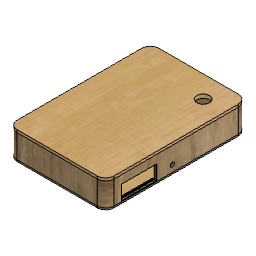
Wildfire prediction Device Full (Autodesk Fusion 360 design; units mm, degrees)
Autodesk Fusion 360 part; units mm, degrees
note: some values were not read from the file. Set by a fixed rule: which sketch regions a step uses.
(part 1 of 2)
sketch "PCB_wildfire-prediction-system_2026-03-05" plane through (0, 0, 0) normal (0, 0, 1) x (1, 0, 0)
  line L0 (72.8848, 47.7095) -> (75.6366, 50.4613)
  line L1 (75.6366, 56.1675) -> (78.2188, 58.7496)
  line L2 (75.6366, 50.4613) -> (75.6366, 56.1675)
  line L3 (93.0849, 97.6657) -> (85.1296, 89.7104)
  line L4 (85.1296, 60.3265) -> (83.9338, 59.1306)
  line L5 (85.1296, 89.7104) -> (85.1296, 60.3265)
  line L6 (79.3633, 25.6026) -> (79.2348, 25.6026)
  line L7 (80.6432, 26.8825) -> (79.3633, 25.6026)
  line L8 (80.6432, 45.1492) -> (80.6432, 26.8825)
  line L9 (78.0918, 47.7006) -> (80.6432, 45.1492)
  line L10 (79.2348, 13.8175) -> (79.2348, 23.0626)
  line L11 (82.5368, 10.5155) -> (79.2348, 13.8175)
  line L12 (83.9338, 61.6706) -> (83.9338, 62.8647)
  line L13 (78.0847, 97.6657) -> (78.0847, 72.6655)
  line L14 (76.5114, 29.9295) -> (72.8848, 29.9295)
  line L15 (79.6288, 33.0469) -> (76.5114, 29.9295)
  line L16 (78.0918, 45.1606) -> (79.6288, 43.6237)
  line L17 (79.6288, 43.6237) -> (79.6288, 33.0469)
  line L18 (76.5114, 25.786) -> (79.2348, 23.0626)
  line L19 (76.5114, 29.9295) -> (76.5114, 25.786)
  line L20 (60.0786, 69.2292) -> (57.3151, 66.4656)
  line L21 (78.0847, 69.2292) -> (60.0786, 69.2292)
  line L22 (78.0847, 68.7138) -> (78.0847, 69.2292)
  line L23 (83.9338, 62.8647) -> (78.0847, 68.7138)
  line L24 (78.0847, 69.2292) -> (78.0847, 72.6655)
  line L25 (72.3605, 36.2795) -> (71.6135, 37.0265)
  line L26 (76.8307, 36.2795) -> (72.3605, 36.2795)
  line L27 (71.6135, 37.0265) -> (71.6135, 54.0582)
  line L28 (78.0918, 37.5406) -> (76.8307, 36.2795)
  line L29 (71.6135, 54.0582) -> (72.8848, 55.3295)
  line L30 (83.9338, 54.0506) -> (81.9043, 54.0506)
  line L31 (74.1909, 41.3956) -> (72.8848, 40.0895)
  line L32 (81.9043, 54.0506) -> (74.1909, 46.3371)
  line L33 (74.1909, 46.3371) -> (74.1909, 41.3956)
  line L34 (24.2753, 76.6251) -> (24.2753, 60.759)
  line L35 (24.2753, 60.759) -> (50.0248, 35.0095)
  line L36 (18.1478, 82.7526) -> (24.2753, 76.6251)
  line L37 (27.021, 60.5533) -> (50.0248, 37.5495)
  line L38 (27.021, 76.4194) -> (27.021, 60.5533)
  line L39 (18.1478, 85.2926) -> (27.021, 76.4194)
  line L40 (51.3293, 31.9107) -> (51.3293, 43.865)
  line L41 (49.4325, 31.1995) -> (50.6181, 31.1995)
  line L42 (41.6428, 4.3936) -> (41.6428, 23.4098)
  line L43 (41.6428, 23.4098) -> (49.4325, 31.1995)
  line L44 (50.6181, 31.1995) -> (51.3293, 31.9107)
  line L45 (51.3293, 43.865) -> (50.0248, 45.1695)
  line L46 (50.5173, 26.1195) -> (49.3784, 26.1195)
  line L47 (51.8815, 27.4837) -> (50.5173, 26.1195)
  line L48 (50.0248, 47.7095) -> (51.8815, 45.8528)
  line L49 (51.8815, 45.8528) -> (51.8815, 27.4837)
  line L50 (49.3784, 26.1195) -> (44.1828, 20.9239)
  line L51 (44.1828, 20.9239) -> (44.1828, 4.3936)
  line L52 (59.8551, 60.0798) -> (50.0248, 50.2495)
  line L53 (59.8551, 66.4656) -> (59.8551, 60.0798)
  line L54 (93.0849, 27.6638) -> (93.0849, 72.6655)
  line L55 (82.5368, 17.1157) -> (93.0849, 27.6638)
  line L56 (-0.1656, 4.5206) -> (-0.1656, 98.5006)
  line L57 (97.6244, 0.7106) -> (3.6444, 0.7106)
  line L58 (101.4344, 98.5006) -> (101.4344, 4.5206)
  line L59 (3.6444, 102.3106) -> (97.6244, 102.3106)
  arc A0 (101.4344, 98.5006) -> (97.6244, 102.3106) centre (97.6244, 98.5006) ccw
  arc A1 (97.6244, 0.7106) -> (101.4344, 4.5206) centre (97.6244, 4.5206) ccw
  arc A2 (-0.1656, 4.5206) -> (3.6444, 0.7106) centre (3.6444, 4.5206) ccw
  arc A3 (3.6444, 102.3106) -> (-0.1656, 98.5006) centre (3.6444, 98.5006) ccw
  line L60 (76.3049, 61.2896) -> (72.8848, 57.8695)
  line L61 (78.2188, 61.2896) -> (76.3049, 61.2896)
  line L62 (45.5572, 56.3242) -> (45.5572, 52.8619)
  line L63 (45.5572, 52.8619) -> (49.4381, 48.981)
  line L64 (46.4688, 57.2358) -> (45.5572, 56.3242)
  line L65 (66.5333, 48.981) -> (72.8848, 42.6295)
  line L66 (49.4381, 48.981) -> (66.5333, 48.981)
  line L67 (54.976, 43.8995) -> (49.325, 43.8995)
  line L68 (74.2716, 42.1599) -> (73.4713, 41.3595)
  line L69 (72.8848, 45.1695) -> (72.8848, 44.6902)
  line L70 (49.325, 43.8995) -> (45.1165, 48.108)
  line L71 (57.516, 41.3595) -> (54.976, 43.8995)
  line L72 (73.4713, 41.3595) -> (57.516, 41.3595)
  line L73 (45.1165, 58.3836) -> (46.4688, 59.7359)
  line L74 (72.8848, 44.6902) -> (74.2716, 43.3034)
  line L75 (45.1165, 48.108) -> (45.1165, 58.3836)
  line L76 (74.2716, 43.3034) -> (74.2716, 42.1599)
  line L77 (74.8983, 31.1995) -> (77.9551, 28.1426)
  line L78 (50.0248, 42.6295) -> (61.4548, 31.1995)
  line L79 (61.4548, 31.1995) -> (74.8983, 31.1995)
  line L80 (79.2348, 28.1426) -> (77.9551, 28.1426)
  line L81 (73.532, 46.4395) -> (72.3562, 46.4395)
  line L82 (78.0918, 40.0806) -> (74.5457, 43.6267)
  line L83 (74.5457, 45.4258) -> (73.532, 46.4395)
  line L84 (74.5457, 43.6267) -> (74.5457, 45.4258)
  line L85 (72.3562, 46.4395) -> (71.5787, 47.217)
  line L86 (71.5787, 51.4834) -> (72.8848, 52.7895)
  line L87 (71.5787, 47.217) -> (71.5787, 51.4834)
  line L88 (78.0918, 42.6206) -> (75.9592, 44.7532)
  line L89 (75.9592, 44.7532) -> (75.9592, 47.1751)
  line L90 (75.9592, 47.1751) -> (72.8848, 50.2495)
  line L91 (78.0918, 47.7006) -> (78.0918, 49.1073)
  line L92 (78.4728, 53.6696) -> (78.2188, 53.6696)
  line L93 (83.9338, 59.1306) -> (78.4728, 53.6696)
  line L94 (78.2188, 53.6696) -> (78.2188, 49.2343)
  line L95 (78.2188, 49.2343) -> (78.0918, 49.1073)
  line L96 (57.5737, 6.0441) -> (77.1322, 25.6026)
  line L97 (38.2133, 6.0441) -> (57.5737, 6.0441)
  line L98 (77.1322, 25.6026) -> (79.2348, 25.6026)
  line L99 (36.5628, 4.3936) -> (38.2133, 6.0441)
  line L100 (85.1296, 60.3265) -> (83.9338, 59.1306)
  line L101 (64.9351, 66.4656) -> (67.2272, 64.1735)
  line L102 (85.1296, 62.7867) -> (85.1296, 60.3265)
  line L103 (83.7428, 64.1735) -> (85.1296, 62.7867)
  line L104 (67.2272, 64.1735) -> (83.7428, 64.1735)
  line L105 (18.1478, 80.2126) -> (47.9202, 80.2126)
  line L106 (47.9202, 80.2126) -> (61.1251, 67.0077)
  line L107 (64.9351, 66.4656) -> (63.576, 67.8248)
  line L108 (63.576, 67.8248) -> (61.9422, 67.8248)
  line L109 (61.9422, 67.8248) -> (61.1251, 67.0077)
  line L110 (49.7591, 59.5708) -> (48.2615, 58.0732)
  line L111 (46.6537, 55.9858) -> (46.4688, 55.9858)
  line L112 (61.1251, 65.9317) -> (54.7642, 59.5708)
  line L113 (48.2615, 57.5937) -> (46.6537, 55.9858)
  line L114 (48.2615, 58.0732) -> (48.2615, 57.5937)
  line L115 (61.1251, 67.0077) -> (61.1251, 65.9317)
  line L116 (54.7642, 59.5708) -> (49.7591, 59.5708)
  line L117 (83.9338, 61.6706) -> (82.7397, 61.6706)
  line L118 (82.5368, 10.5155) -> (83.4367, 10.5155)
  line L119 (83.4367, 10.5155) -> (87.0369, 14.1157)
  line L120 (82.7397, 61.6706) -> (82.7397, 60.7306)
  line L121 (82.7397, 60.7306) -> (78.2188, 56.2096)
  line L122 (76.4946, 54.4855) -> (76.4946, 46.5713)
  line L123 (78.2188, 56.2096) -> (76.4946, 54.4855)
  line L124 (76.4946, 46.5713) -> (77.9054, 45.1606)
  line L125 (77.9054, 45.1606) -> (78.0918, 45.1606)
  line L126 (35.4536, 2.9628) -> (34.0228, 4.3936)
  line L127 (37.672, 2.9628) -> (35.4536, 2.9628)
  line L128 (39.1028, 4.3936) -> (37.672, 2.9628)
  line L129 (39.1028, 4.3936) -> (40.5194, 2.9771)
  line L130 (40.5194, 2.9771) -> (74.9983, 2.9771)
  line L131 (74.9983, 2.9771) -> (82.5368, 10.5155)
  line L132 (57.3151, 66.4656) -> (53.9417, 63.0923)
  line L133 (53.9417, 63.0923) -> (46.4688, 63.0923)
  line L134 (46.4688, 62.2355) -> (46.4688, 63.0923)
  line L135 (18.1478, 77.6726) -> (31.8884, 77.6726)
  line L136 (31.8884, 77.6726) -> (46.4688, 63.0923)
  line L137 (78.7583, 36.2434) -> (74.1909, 36.2434)
  line L138 (83.9338, 56.5906) -> (79.5747, 52.2315)
  line L139 (79.5747, 52.2315) -> (79.5747, 37.0598)
  line L140 (79.5747, 37.0598) -> (78.7583, 36.2434)
  line L141 (74.1909, 36.2434) -> (72.8848, 37.5495)
  line L142 (62.3951, 65.1598) -> (50.0248, 52.7895)
  line L143 (62.3951, 66.4656) -> (62.3951, 65.1598)
  line L144 (47.7387, 63.8297) -> (47.7387, 52.0187)
  line L145 (44.4367, 63.8297) -> (47.7387, 63.8297)
  line L146 (44.4367, 51.8917) -> (44.4367, 63.8297)
  line L147 (47.7387, 51.8917) -> (44.4367, 51.8917)
  line L148 (2.8371, 13.6149) -> (40.838, 13.6149)
  line L149 (40.838, 63.6148) -> (2.8371, 63.6148)
  line L150 (40.838, 13.6149) -> (40.838, 63.6148)
  line L151 (2.8371, 63.6148) -> (2.8371, 13.6149)
  line L152 (42.8378, 19.6157) -> (40.838, 19.6157)
  line L153 (42.8378, 19.6157) -> (42.8378, 38.6158)
  line L154 (42.8378, 38.6158) -> (40.838, 38.6158)
  line L155 (2.8371, 36.1167) -> (0.3378, 36.1167)
  line L156 (0.3378, 21.1156) -> (2.8371, 21.1156)
  line L157 (2.8379, 36.1156) -> (2.8371, 36.1167)
  line L158 (0.3378, 36.1167) -> (0.3378, 21.1156)
  line L159 (91.4626, 33.3886) -> (91.4626, 19.0376)
  line L160 (91.4626, 19.0376) -> (76.4847, 19.0376)
  line L161 (76.4847, 19.0376) -> (76.4847, 33.3886)
  line L162 (76.4847, 33.3886) -> (91.4626, 33.3886)
  line L163 (48.7548, 62.8698) -> (74.1548, 62.8698)
  line L164 (48.7548, 2.8696) -> (48.7548, 62.8698)
  line L165 (74.1548, 62.8698) -> (74.1548, 2.8696)
  line L166 (74.1548, 2.8696) -> (48.7548, 2.8696)
  line L167 (56.8109, 96.1056) -> (54.1109, 96.1056)
  line L168 (56.8109, 98.7056) -> (56.8109, 96.1056)
  line L169 (54.1109, 96.1056) -> (54.1109, 98.7056)
  line L170 (54.1109, 98.7056) -> (56.8109, 98.7056)
  line L171 (47.8209, 100.4056) -> (47.8209, 64.8057)
  line L172 (73.9008, 64.8057) -> (73.9008, 100.4056)
  line L173 (47.8209, 64.8057) -> (73.9008, 64.8057)
  line L174 (73.9008, 100.4056) -> (47.8209, 100.4056)
  line L175 (32.4988, 2.6156) -> (32.4988, 6.1716)
  line L176 (45.7068, 2.6156) -> (32.4988, 2.6156)
  line L177 (32.4988, 6.1716) -> (45.7068, 6.1716)
  line L178 (45.7068, 6.1716) -> (45.7068, 2.6156)
  line L179 (77.3298, 43.8906) -> (76.8218, 44.3986)
  line L180 (77.3298, 41.3506) -> (76.8218, 41.8586)
  line L181 (76.8218, 43.3826) -> (77.3298, 43.8906)
  line L182 (76.8218, 46.9386) -> (76.8218, 48.9706)
  line L183 (76.8218, 39.3186) -> (76.8218, 40.8426)
  line L184 (76.8218, 36.2706) -> (76.8218, 38.3026)
  line L185 (76.8218, 41.8586) -> (76.8218, 43.3826)
  line L186 (76.8218, 38.3026) -> (77.3298, 38.8106)
  line L187 (79.3618, 38.3026) -> (79.3618, 36.2706)
  line L188 (78.8538, 43.8906) -> (79.3618, 43.3826)
  line L189 (76.8218, 45.9226) -> (77.3298, 46.4306)
  line L190 (79.3618, 44.3986) -> (78.8538, 43.8906)
  line L191 (79.3618, 40.8426) -> (79.3618, 39.3186)
  line L192 (79.3618, 41.8586) -> (78.8538, 41.3506)
  line L193 (79.3618, 43.3826) -> (79.3618, 41.8586)
  line L194 (76.8218, 48.9706) -> (79.3618, 48.9706)
  line L195 (76.8218, 44.3986) -> (76.8218, 45.9226)
  line L196 (77.3298, 38.8106) -> (76.8218, 39.3186)
  line L197 (78.8538, 46.4306) -> (79.3618, 45.9226)
  line L198 (77.3298, 46.4306) -> (76.8218, 46.9386)
  line L199 (79.3618, 48.9706) -> (79.3618, 46.9386)
  line L200 (79.3618, 36.2706) -> (76.8218, 36.2706)
  line L201 (76.8218, 40.8426) -> (77.3298, 41.3506)
  line L202 (79.3618, 46.9386) -> (78.8538, 46.4306)
  line L203 (79.3618, 45.9226) -> (79.3618, 44.3986)
  line L204 (78.8538, 41.3506) -> (79.3618, 40.8426)
  line L205 (79.3618, 39.3186) -> (78.8538, 38.8106)
  line L206 (78.8538, 38.8106) -> (79.3618, 38.3026)
  line L207 (76.3918, 50.1507) -> (99.1919, 50.1507)
  line L208 (99.1738, 35.0006) -> (99.1738, 34.9836)
  line L209 (99.1738, 42.6206) -> (99.1738, 35.0006)
  line L210 (99.1738, 50.1136) -> (99.1738, 42.6206)
  line L211 (99.1738, 35.0006) -> (76.3918, 35.0006)
  line L212 (76.3138, 35.0006) -> (76.3138, 50.1136)
  line L213 (92.9508, 42.6206) -> (92.9508, 45.1207)
  line L214 (92.9508, 40.1208) -> (92.9508, 42.6206)
  line L215 (85.9658, 45.1606) -> (85.9508, 45.1606)
  line L216 (92.9508, 45.1606) -> (85.9658, 45.1606)
  line L217 (85.9658, 45.1606) -> (85.9658, 40.1208)
  line L218 (92.9508, 40.0806) -> (85.9658, 40.0806)
  line L219 (75.5848, 100.1656) -> (95.5848, 100.1656)
  line L220 (95.5848, 100.1656) -> (95.5848, 70.1657)
  line L221 (95.5848, 70.1657) -> (75.5848, 70.1657)
  line L222 (75.5848, 70.1657) -> (75.5848, 100.1656)
  line L223 (16.8778, 95.1986) -> (44.8178, 95.1986)
  line L224 (44.8178, 73.8626) -> (44.8178, 67.7666)
  line L225 (16.8778, 67.7666) -> (16.8778, 95.1986)
  line L226 (44.8178, 89.1026) -> (44.8178, 73.8626)
  line L227 (44.8178, 95.1986) -> (44.8178, 89.1026)
  line L228 (44.8178, 67.7666) -> (16.8778, 67.7666)
  line L229 (19.4178, 78.3076) -> (19.4178, 77.0376)
  line L230 (19.4178, 79.5776) -> (18.7828, 78.9426)
  line L231 (16.8778, 85.9276) -> (17.5128, 86.5626)
  line L232 (18.7828, 86.5626) -> (19.4178, 85.9276)
  line L233 (18.7828, 81.4826) -> (19.4178, 80.8476)
  line L234 (18.7828, 84.0226) -> (19.4178, 83.3876)
  line L235 (18.7828, 76.4026) -> (17.5128, 76.4026)
  line L236 (19.4178, 83.3876) -> (19.4178, 82.1176)
  line L237 (19.4178, 80.8476) -> (19.4178, 79.5776)
  line L238 (19.4178, 82.1176) -> (18.7828, 81.4826)
  line L239 (17.5128, 86.5626) -> (18.7828, 86.5626)
  line L240 (19.4178, 85.9276) -> (19.4178, 84.6576)
  line L241 (18.7828, 78.9426) -> (19.4178, 78.3076)
  line L242 (19.4178, 84.6576) -> (18.7828, 84.0226)
  line L243 (19.4178, 77.0376) -> (18.7828, 76.4026)
  line L244 (17.5128, 76.4026) -> (16.8778, 77.0376)
  line L245 (17.5128, 78.9426) -> (16.8778, 79.5776)
  line L246 (16.8778, 78.3076) -> (17.5128, 78.9426)
  line L247 (16.8778, 80.8476) -> (17.5128, 81.4826)
  line L248 (17.5128, 81.4826) -> (16.8778, 82.1176)
  line L249 (17.5128, 84.0226) -> (16.8778, 84.6576)
  line L250 (16.8778, 83.3876) -> (17.5128, 84.0226)
  line L251 (22.7198, 92.9126) -> (36.4358, 92.9126)
  line L252 (22.7198, 70.0526) -> (22.7198, 92.9126)
  line L253 (36.4358, 92.9126) -> (36.4358, 70.0526)
  line L254 (36.4358, 70.0526) -> (22.7198, 70.0526)
  line L255 (20.8148, 80.2126) -> (19.7988, 80.2126)
  line L256 (20.8148, 85.2926) -> (19.7988, 85.2926)
  line L257 (44.8178, 73.8626) -> (42.9128, 75.1326)
  line L258 (42.9128, 87.8326) -> (44.8178, 89.1026)
  line L259 (42.9128, 75.1326) -> (42.9128, 87.8326)
  line L260 (79.4888, 62.5596) -> (79.4888, 52.3996)
  line L261 (76.9488, 52.3996) -> (76.9488, 62.5596)
  line L262 (76.9488, 62.5596) -> (79.4888, 62.5596)
  line L263 (79.4888, 52.3996) -> (76.9488, 52.3996)
  line L264 (88.5368, 2.6156) -> (76.5368, 2.6156)
  line L265 (88.5368, 18.1157) -> (88.5368, 2.6156)
  line L266 (76.5368, 18.1157) -> (88.5368, 18.1157)
  line L267 (76.5368, 2.6156) -> (76.5368, 18.1157)
  line L268 (82.6638, 52.7806) -> (82.6638, 62.9406)
  line L269 (85.2038, 62.9406) -> (85.2038, 61.0356)
  line L270 (82.6638, 62.9406) -> (85.2038, 62.9406)
  line L271 (85.2038, 52.7806) -> (82.6638, 52.7806)
  line L272 (85.2038, 52.7806) -> (85.2038, 61.0356)
  arc A4 (97.4982, 46.8116) -> (97.4918, 46.6671) centre (95.8718, 46.8107) ccw
  arc A5 (97.4631, 38.3026) -> (97.4568, 38.1611) centre (95.8718, 38.3032) ccw
  circle A6 centre (38.3408, 16.0078) radius 1.2499
  circle A7 centre (5.3208, 16.0078) radius 1.2499
  circle A8 centre (38.3408, 61.2198) radius 1.2499
  circle A9 centre (5.3208, 60.9658) radius 1.2499
  line L273 (79.9968, 63.0676) -> (76.4408, 63.0676)
  line L274 (80.0189, 51.8695) -> (79.9968, 63.0676)
  line L275 (76.4187, 51.8695) -> (80.0189, 51.8695)
  line L276 (76.4408, 63.0676) -> (76.4187, 51.8695)
  line L277 (79.4888, 62.5596) -> (79.4888, 53.0346)
  line L278 (78.8538, 52.3996) -> (76.9488, 52.3996)
  line L279 (79.4888, 53.0346) -> (78.8538, 52.3996)
  line L280 (76.9488, 62.5596) -> (79.4888, 62.5596)
  line L281 (76.9488, 52.3996) -> (76.9488, 62.5596)
  circle A10 centre (46.4687, 53.4855) radius 0.3839
  circle A11 centre (46.4688, 53.4857) radius 0.5758
  circle A12 centre (46.4687, 54.7355) radius 0.3839
  circle A13 centre (46.4688, 54.7357) radius 0.5758
  circle A14 centre (46.4687, 55.9857) radius 0.3839
  circle A15 centre (46.4688, 55.9858) radius 0.5758
  circle A16 centre (46.4687, 57.2356) radius 0.3839
  circle A17 centre (46.4688, 57.2358) radius 0.5758
  circle A18 centre (46.4687, 58.4855) radius 0.3839
  circle A19 centre (46.4688, 58.4857) radius 0.5758
  circle A20 centre (46.4687, 59.7357) radius 0.3839
  circle A21 centre (46.4688, 59.7359) radius 0.5758
  circle A22 centre (46.4687, 60.9857) radius 0.3839
  circle A23 centre (46.4688, 60.9858) radius 0.5758
  circle A24 centre (46.4687, 62.2356) radius 0.3895
  circle A25 centre (79.2348, 23.0626) radius 0.6305
  circle A26 centre (79.2349, 25.6025) radius 0.6305
  circle A27 centre (79.2348, 25.6026) radius 1.0508
  circle A28 centre (79.2348, 28.1426) radius 0.6305
  circle A29 centre (72.8849, 57.8696) radius 0.4816
  circle A30 centre (72.8848, 57.8695) radius 1.0033
  circle A31 centre (72.8849, 55.3296) radius 0.4816
  circle A32 centre (72.8848, 55.3295) radius 1.0033
  circle A33 centre (72.8849, 52.7896) radius 0.4816
  circle A34 centre (72.8848, 52.7895) radius 1.0033
  circle A35 centre (72.8849, 50.2496) radius 0.4816
  circle A36 centre (72.8848, 50.2495) radius 1.0033
  circle A37 centre (72.8849, 47.7096) radius 0.4816
  circle A38 centre (72.8848, 47.7095) radius 1.0033
  circle A39 centre (72.8849, 45.1696) radius 0.4816
  circle A40 centre (72.8848, 45.1695) radius 1.0033
  circle A41 centre (72.8849, 42.6296) radius 0.4816
  circle A42 centre (72.8848, 42.6295) radius 1.0033
  circle A43 centre (72.8849, 40.0896) radius 0.4816
  circle A44 centre (72.8848, 40.0895) radius 1.0033
  circle A45 centre (72.8849, 37.5496) radius 0.4816
  circle A46 centre (72.8848, 37.5495) radius 1.0033
  circle A47 centre (72.8849, 35.0096) radius 0.4816
  circle A48 centre (72.8848, 35.0095) radius 1.0033
  circle A49 centre (72.8849, 32.4696) radius 0.4816
  circle A50 centre (72.8848, 32.4695) radius 1.0033
  circle A51 centre (72.8849, 29.9296) radius 0.4816
  circle A52 centre (72.8848, 29.9295) radius 1.0033
  circle A53 centre (72.8849, 27.3896) radius 0.4816
  circle A54 centre (72.8848, 27.3895) radius 1.0033
  circle A55 centre (72.8849, 24.8496) radius 0.4816
  circle A56 centre (72.8848, 24.8495) radius 1.0033
  circle A57 centre (50.0249, 14.6896) radius 0.4816
  circle A58 centre (50.0248, 14.6895) radius 1.0033
  circle A59 centre (50.0249, 17.2296) radius 0.4816
  circle A60 centre (50.0248, 17.2295) radius 1.0033
  circle A61 centre (50.0249, 19.7696) radius 0.4816
  circle A62 centre (50.0248, 19.7695) radius 1.0033
  circle A63 centre (50.0249, 22.3096) radius 0.4816
  circle A64 centre (50.0248, 22.3095) radius 1.0033
  circle A65 centre (50.0249, 24.8496) radius 0.4816
  circle A66 centre (50.0248, 24.8495) radius 1.0033
  circle A67 centre (50.0249, 27.3896) radius 0.4816
  circle A68 centre (50.0248, 27.3895) radius 1.0033
  circle A69 centre (50.0249, 29.9296) radius 0.4816
  circle A70 centre (50.0248, 29.9295) radius 1.0033
  circle A71 centre (50.0249, 32.4696) radius 0.4816
  circle A72 centre (50.0248, 32.4695) radius 1.0033
  circle A73 centre (50.0249, 35.0096) radius 0.4816
  circle A74 centre (50.0248, 35.0095) radius 1.0033
  circle A75 centre (50.0249, 37.5496) radius 0.4816
  circle A76 centre (50.0248, 37.5495) radius 1.0033
  circle A77 centre (50.0249, 40.0896) radius 0.4816
  circle A78 centre (50.0248, 40.0895) radius 1.0033
  circle A79 centre (50.0249, 42.6296) radius 0.4816
  circle A80 centre (50.0248, 42.6295) radius 1.0033
  circle A81 centre (50.0249, 45.1696) radius 0.4816
  circle A82 centre (50.0248, 45.1695) radius 1.0033
  circle A83 centre (50.0249, 47.7096) radius 0.4816
  circle A84 centre (50.0248, 47.7095) radius 1.0033
  circle A85 centre (50.0249, 50.2496) radius 0.4816
  circle A86 centre (50.0248, 50.2495) radius 1.0033
  circle A87 centre (50.0249, 52.7896) radius 0.4816
  circle A88 centre (50.0248, 52.7895) radius 1.0033
  circle A89 centre (50.0249, 55.3296) radius 0.4816
  circle A90 centre (50.0248, 55.3295) radius 1.0033
  circle A91 centre (50.0249, 57.8696) radius 0.4816
  circle A92 centre (50.0248, 57.8695) radius 1.0033
  circle A93 centre (64.935, 66.4657) radius 0.5334
  circle A94 centre (64.9351, 66.4656) radius 0.889
  circle A95 centre (62.395, 66.4657) radius 0.5334
  circle A96 centre (62.3951, 66.4656) radius 0.889
  circle A97 centre (59.855, 66.4657) radius 0.5334
  circle A98 centre (59.8551, 66.4656) radius 0.889
  circle A99 centre (57.315, 66.4657) radius 0.5334
  circle A100 centre (57.3151, 66.4656) radius 0.889
  circle A101 centre (34.0228, 4.3936) radius 0.5127
  circle A102 centre (34.0228, 4.3936) radius 1.0254
  circle A103 centre (36.5628, 4.3936) radius 0.5127
  circle A104 centre (36.5628, 4.3936) radius 1.0254
  circle A105 centre (39.1028, 4.3936) radius 0.5127
  circle A106 centre (39.1028, 4.3936) radius 1.0254
  circle A107 centre (41.6428, 4.3936) radius 0.5127
  circle A108 centre (41.6428, 4.3936) radius 1.0254
  circle A109 centre (44.1828, 4.3936) radius 0.5127
  circle A110 centre (44.1828, 4.3936) radius 1.0254
  arc A111 (78.0917, 48.2132) -> (78.0917, 47.1881) centre (78.0917, 47.7006) ccw
  arc A112 (78.092, 47.1881) -> (78.092, 48.2132) centre (78.092, 47.7006) ccw
  line L282 (78.0917, 48.2132) -> (78.092, 48.2132)
  line L283 (78.092, 48.2132) -> (78.0917, 48.2132)
  line L284 (78.0917, 47.1881) -> (78.092, 47.1881)
  line L285 (78.092, 47.1881) -> (78.0917, 47.1881)
  circle A113 centre (78.0918, 45.1606) radius 1.0254
  arc A114 (78.0917, 45.6732) -> (78.0917, 44.6481) centre (78.0917, 45.1606) ccw
  arc A115 (78.092, 44.6481) -> (78.092, 45.6732) centre (78.092, 45.1606) ccw
  line L286 (78.0917, 45.6732) -> (78.092, 45.6732)
  line L287 (78.092, 45.6732) -> (78.0917, 45.6732)
  line L288 (78.0917, 44.6481) -> (78.092, 44.6481)
  line L289 (78.092, 44.6481) -> (78.0917, 44.6481)
  circle A116 centre (78.0918, 42.6206) radius 1.0254
  arc A117 (78.0917, 43.1332) -> (78.0917, 42.1081) centre (78.0917, 42.6206) ccw
  arc A118 (78.092, 42.1081) -> (78.092, 43.1332) centre (78.092, 42.6206) ccw
  line L290 (78.092, 43.1332) -> (78.0917, 43.1332)
  line L291 (78.0917, 43.1332) -> (78.092, 43.1332)
  line L292 (78.0917, 42.1081) -> (78.092, 42.1081)
  line L293 (78.092, 42.1081) -> (78.0917, 42.1081)
  circle A119 centre (78.0918, 40.0806) radius 1.0254
  arc A120 (78.0917, 40.5932) -> (78.0917, 39.5681) centre (78.0917, 40.0806) ccw
  arc A121 (78.092, 39.5681) -> (78.092, 40.5932) centre (78.092, 40.0806) ccw
  line L294 (78.092, 40.5932) -> (78.0917, 40.5932)
  line L295 (78.0917, 40.5932) -> (78.092, 40.5932)
  line L296 (78.092, 39.5681) -> (78.0917, 39.5681)
  line L297 (78.0917, 39.5681) -> (78.092, 39.5681)
  circle A122 centre (78.0918, 37.5406) radius 1.0254
  arc A123 (78.0917, 38.0532) -> (78.0917, 37.0281) centre (78.0917, 37.5406) ccw
  arc A124 (78.092, 37.0281) -> (78.092, 38.0532) centre (78.092, 37.5406) ccw
  line L298 (78.0917, 38.0532) -> (78.092, 38.0532)
  line L299 (78.092, 38.0532) -> (78.0917, 38.0532)
  line L300 (78.092, 37.0281) -> (78.0917, 37.0281)
  line L301 (78.0917, 37.0281) -> (78.092, 37.0281)
  circle A125 centre (78.0847, 72.6655) radius 0.4732
  circle A126 centre (78.0847, 72.6655) radius 0.8383
  circle A127 centre (78.0847, 97.6657) radius 0.4732
  circle A128 centre (78.0847, 97.6657) radius 0.8383
  circle A129 centre (93.0849, 97.6657) radius 0.4732
  circle A130 centre (93.0849, 97.6657) radius 0.8383
  circle A131 centre (93.0849, 72.6655) radius 0.4732
  circle A132 centre (93.0849, 72.6655) radius 0.8383
  arc A133 (17.6311, 77.6725) -> (18.6645, 77.6725) centre (18.1478, 77.6725) ccw
  arc A134 (18.6645, 77.6728) -> (17.6311, 77.6728) centre (18.1478, 77.6728) ccw
  line L302 (17.6311, 77.6725) -> (17.6311, 77.6728)
  line L303 (17.6311, 77.6728) -> (17.6311, 77.6725)
  line L304 (18.6645, 77.6725) -> (18.6645, 77.6728)
  line L305 (18.6645, 77.6728) -> (18.6645, 77.6725)
  circle A135 centre (18.1478, 80.2126) radius 0.7794
  arc A136 (17.6311, 80.2125) -> (18.6645, 80.2125) centre (18.1478, 80.2125) ccw
  arc A137 (18.6645, 80.2128) -> (17.6311, 80.2128) centre (18.1478, 80.2128) ccw
  line L306 (17.6311, 80.2128) -> (17.6311, 80.2125)
  line L307 (17.6311, 80.2125) -> (17.6311, 80.2128)
  line L308 (18.6645, 80.2125) -> (18.6645, 80.2128)
  line L309 (18.6645, 80.2128) -> (18.6645, 80.2125)
  circle A138 centre (18.1478, 82.7526) radius 0.7794
  arc A139 (17.6311, 82.7525) -> (18.6645, 82.7525) centre (18.1478, 82.7525) ccw
  arc A140 (18.6645, 82.7528) -> (17.6311, 82.7528) centre (18.1478, 82.7528) ccw
  line L310 (17.6311, 82.7528) -> (17.6311, 82.7525)
  line L311 (17.6311, 82.7525) -> (17.6311, 82.7528)
  line L312 (18.6645, 82.7525) -> (18.6645, 82.7528)
  line L313 (18.6645, 82.7528) -> (18.6645, 82.7525)
  circle A141 centre (18.1478, 85.2926) radius 0.7794
  arc A142 (17.6311, 85.2925) -> (18.6645, 85.2925) centre (18.1478, 85.2925) ccw
  arc A143 (18.6645, 85.2928) -> (17.6311, 85.2928) centre (18.1478, 85.2928) ccw
  line L314 (17.6311, 85.2928) -> (17.6311, 85.2925)
  line L315 (17.6311, 85.2925) -> (17.6311, 85.2928)
  line L316 (18.6645, 85.2925) -> (18.6645, 85.2928)
  line L317 (18.6645, 85.2928) -> (18.6645, 85.2925)
  arc A144 (78.2443, 58.2395) -> (78.2443, 59.2598) centre (78.2443, 58.7496) ccw
  arc A145 (78.1933, 59.2598) -> (78.1933, 58.2395) centre (78.1933, 58.7496) ccw
  line L318 (78.1933, 58.2395) -> (78.2443, 58.2395)
  line L319 (78.2443, 58.2395) -> (78.1933, 58.2395)
  line L320 (78.2443, 59.2598) -> (78.1933, 59.2598)
  line L321 (78.1933, 59.2598) -> (78.2443, 59.2598)
  arc A146 (78.2443, 55.6995) -> (78.2443, 56.7198) centre (78.2443, 56.2096) ccw
  arc A147 (78.1933, 56.7198) -> (78.1933, 55.6995) centre (78.1933, 56.2096) ccw
  line L322 (78.1933, 55.6995) -> (78.2443, 55.6995)
  line L323 (78.2443, 55.6995) -> (78.1933, 55.6995)
  line L324 (78.2443, 56.7198) -> (78.1933, 56.7198)
  line L325 (78.1933, 56.7198) -> (78.2443, 56.7198)
  arc A148 (78.2443, 53.1595) -> (78.2443, 54.1798) centre (78.2443, 53.6696) ccw
  arc A149 (78.1933, 54.1798) -> (78.1933, 53.1595) centre (78.1933, 53.6696) ccw
  line L326 (78.2443, 53.1595) -> (78.1933, 53.1595)
  line L327 (78.1933, 53.1595) -> (78.2443, 53.1595)
  line L328 (78.1933, 54.1798) -> (78.2443, 54.1798)
  line L329 (78.2443, 54.1798) -> (78.1933, 54.1798)
  arc A150 (78.2443, 60.7795) -> (78.2443, 61.7998) centre (78.2443, 61.2896) ccw
  arc A151 (78.1933, 61.7998) -> (78.1933, 60.7795) centre (78.1933, 61.2896) ccw
  line L330 (78.2443, 60.7795) -> (78.1933, 60.7795)
  line L331 (78.1933, 60.7795) -> (78.2443, 60.7795)
  line L332 (78.1933, 61.7998) -> (78.2443, 61.7998)
  line L333 (78.2443, 61.7998) -> (78.1933, 61.7998)
  arc A152 (81.3711, 16.4798) -> (81.3711, 17.7515) centre (81.3711, 17.1156) ccw
  arc A153 (83.7026, 17.7515) -> (83.7026, 16.4798) centre (83.7026, 17.1156) ccw
  line L334 (81.3711, 16.4798) -> (83.7026, 16.4798)
  line L335 (83.7026, 16.4798) -> (81.3711, 16.4798)
  line L336 (83.7026, 17.7515) -> (81.3711, 17.7515)
  line L337 (81.3711, 17.7515) -> (83.7026, 17.7515)
  arc A154 (87.6727, 12.9877) -> (86.401, 12.9877) centre (87.0368, 12.9877) ccw
  arc A155 (86.401, 15.2435) -> (87.6727, 15.2435) centre (87.0368, 15.2435) ccw
  line L338 (86.401, 12.9877) -> (86.401, 15.2435)
  line L339 (86.401, 15.2435) -> (86.401, 12.9877)
  line L340 (87.6727, 12.9877) -> (87.6727, 15.2435)
  line L341 (87.6727, 15.2435) -> (87.6727, 12.9877)
  arc A156 (81.404, 9.8977) -> (81.404, 11.1336) centre (81.404, 10.5156) ccw
  arc A157 (83.6697, 11.1336) -> (83.6697, 9.8977) centre (83.6697, 10.5156) ccw
  line L342 (83.6697, 9.8977) -> (81.404, 9.8977)
  line L343 (81.404, 9.8977) -> (83.6697, 9.8977)
  line L344 (81.404, 11.1336) -> (83.6697, 11.1336)
  line L345 (83.6697, 11.1336) -> (81.404, 11.1336)
  circle A158 centre (83.9338, 61.6706) radius 0.4588
  circle A159 centre (83.9338, 59.1306) radius 0.4588
  circle A160 centre (83.9338, 59.1306) radius 0.8128
  circle A161 centre (83.9338, 56.5906) radius 0.4588
  circle A162 centre (83.9338, 56.5906) radius 0.8128
  circle A163 centre (83.9338, 54.0506) radius 0.4588
  circle A164 centre (83.9338, 54.0506) radius 0.8128
  circle A165 centre (46.4687, 53.4855) radius 0.3839
  circle A166 centre (46.4688, 53.4857) radius 0.5758
  circle A167 centre (46.4687, 54.7355) radius 0.3839
  circle A168 centre (46.4688, 54.7357) radius 0.5758
  circle A169 centre (46.4687, 55.9857) radius 0.3839
  circle A170 centre (46.4688, 55.9858) radius 0.5758
  circle A171 centre (46.4687, 57.2356) radius 0.3839
  circle A172 centre (46.4688, 57.2358) radius 0.5758
  circle A173 centre (46.4687, 58.4855) radius 0.3839
  circle A174 centre (46.4688, 58.4857) radius 0.5758
  circle A175 centre (46.4687, 59.7357) radius 0.3839
  circle A176 centre (46.4688, 59.7359) radius 0.5758
  circle A177 centre (46.4687, 60.9857) radius 0.3839
  circle A178 centre (46.4688, 60.9858) radius 0.5758
  circle A179 centre (46.4687, 62.2356) radius 0.3895
  circle A180 centre (79.2348, 23.0626) radius 0.6305
  circle A181 centre (79.2349, 25.6025) radius 0.6305
  circle A182 centre (79.2348, 25.6026) radius 1.0508
  circle A183 centre (79.2348, 28.1426) radius 0.6305
  circle A184 centre (72.8849, 57.8696) radius 0.4816
  circle A185 centre (72.8848, 57.8695) radius 1.0033
  circle A186 centre (72.8849, 55.3296) radius 0.4816
  circle A187 centre (72.8848, 55.3295) radius 1.0033
  circle A188 centre (72.8849, 52.7896) radius 0.4816
  circle A189 centre (72.8848, 52.7895) radius 1.0033
  circle A190 centre (72.8849, 50.2496) radius 0.4816
  circle A191 centre (72.8848, 50.2495) radius 1.0033
  circle A192 centre (72.8849, 47.7096) radius 0.4816
  circle A193 centre (72.8848, 47.7095) radius 1.0033
  circle A194 centre (72.8849, 45.1696) radius 0.4816
  circle A195 centre (72.8848, 45.1695) radius 1.0033
  circle A196 centre (72.8849, 42.6296) radius 0.4816
  circle A197 centre (72.8848, 42.6295) radius 1.0033
  circle A198 centre (72.8849, 40.0896) radius 0.4816
  circle A199 centre (72.8848, 40.0895) radius 1.0033
  circle A200 centre (72.8849, 37.5496) radius 0.4816
  circle A201 centre (72.8848, 37.5495) radius 1.0033
  circle A202 centre (72.8849, 35.0096) radius 0.4816
  circle A203 centre (72.8848, 35.0095) radius 1.0033
  circle A204 centre (72.8849, 32.4696) radius 0.4816
  circle A205 centre (72.8848, 32.4695) radius 1.0033
  circle A206 centre (72.8849, 29.9296) radius 0.4816
  circle A207 centre (72.8848, 29.9295) radius 1.0033
  circle A208 centre (72.8849, 27.3896) radius 0.4816
  circle A209 centre (72.8848, 27.3895) radius 1.0033
  circle A210 centre (72.8849, 24.8496) radius 0.4816
  circle A211 centre (72.8848, 24.8495) radius 1.0033
  circle A212 centre (50.0249, 14.6896) radius 0.4816
  circle A213 centre (50.0248, 14.6895) radius 1.0033
  circle A214 centre (50.0249, 17.2296) radius 0.4816
  circle A215 centre (50.0248, 17.2295) radius 1.0033
  circle A216 centre (50.0249, 19.7696) radius 0.4816
  circle A217 centre (50.0248, 19.7695) radius 1.0033
  circle A218 centre (50.0249, 22.3096) radius 0.4816
  circle A219 centre (50.0248, 22.3095) radius 1.0033
  circle A220 centre (50.0249, 24.8496) radius 0.4816
  circle A221 centre (50.0248, 24.8495) radius 1.0033
  circle A222 centre (50.0249, 27.3896) radius 0.4816
  circle A223 centre (50.0248, 27.3895) radius 1.0033
  circle A224 centre (50.0249, 29.9296) radius 0.4816
  circle A225 centre (50.0248, 29.9295) radius 1.0033
  circle A226 centre (50.0249, 32.4696) radius 0.4816
  circle A227 centre (50.0248, 32.4695) radius 1.0033
  circle A228 centre (50.0249, 35.0096) radius 0.4816
  circle A229 centre (50.0248, 35.0095) radius 1.0033
  circle A230 centre (50.0249, 37.5496) radius 0.4816
  circle A231 centre (50.0248, 37.5495) radius 1.0033
  circle A232 centre (50.0249, 40.0896) radius 0.4816
  circle A233 centre (50.0248, 40.0895) radius 1.0033
  circle A234 centre (50.0249, 42.6296) radius 0.4816
  circle A235 centre (50.0248, 42.6295) radius 1.0033
  circle A236 centre (50.0249, 45.1696) radius 0.4816
  circle A237 centre (50.0248, 45.1695) radius 1.0033
  circle A238 centre (50.0249, 47.7096) radius 0.4816
  circle A239 centre (50.0248, 47.7095) radius 1.0033
  circle A240 centre (50.0249, 50.2496) radius 0.4816
  circle A241 centre (50.0248, 50.2495) radius 1.0033
  circle A242 centre (50.0249, 52.7896) radius 0.4816
  circle A243 centre (50.0248, 52.7895) radius 1.0033
  circle A244 centre (50.0249, 55.3296) radius 0.4816
  circle A245 centre (50.0248, 55.3295) radius 1.0033
  circle A246 centre (50.0249, 57.8696) radius 0.4816
  circle A247 centre (50.0248, 57.8695) radius 1.0033
  circle A248 centre (64.935, 66.4657) radius 0.5334
  circle A249 centre (64.9351, 66.4656) radius 0.889
  circle A250 centre (62.395, 66.4657) radius 0.5334
  circle A251 centre (62.3951, 66.4656) radius 0.889
  circle A252 centre (59.855, 66.4657) radius 0.5334
  circle A253 centre (59.8551, 66.4656) radius 0.889
  circle A254 centre (57.315, 66.4657) radius 0.5334
  circle A255 centre (57.3151, 66.4656) radius 0.889
  circle A256 centre (34.0228, 4.3936) radius 0.5127
  circle A257 centre (34.0228, 4.3936) radius 1.0254
  circle A258 centre (36.5628, 4.3936) radius 0.5127
  circle A259 centre (36.5628, 4.3936) radius 1.0254
  circle A260 centre (39.1028, 4.3936) radius 0.5127
  circle A261 centre (39.1028, 4.3936) radius 1.0254
  circle A262 centre (41.6428, 4.3936) radius 0.5127
  circle A263 centre (41.6428, 4.3936) radius 1.0254
  circle A264 centre (44.1828, 4.3936) radius 0.5127
  circle A265 centre (44.1828, 4.3936) radius 1.0254
  arc A266 (78.0917, 48.2132) -> (78.0917, 47.1881) centre (78.0917, 47.7006) ccw
  arc A267 (78.092, 47.1881) -> (78.092, 48.2132) centre (78.092, 47.7006) ccw
  line L346 (78.092, 48.2132) -> (78.0917, 48.2132)
  line L347 (78.0917, 48.2132) -> (78.092, 48.2132)
  line L348 (78.092, 47.1881) -> (78.0917, 47.1881)
  line L349 (78.0917, 47.1881) -> (78.092, 47.1881)
  circle A268 centre (78.0918, 45.1606) radius 1.0254
  arc A269 (78.0917, 45.6732) -> (78.0917, 44.6481) centre (78.0917, 45.1606) ccw
  arc A270 (78.092, 44.6481) -> (78.092, 45.6732) centre (78.092, 45.1606) ccw
  line L350 (78.092, 45.6732) -> (78.0917, 45.6732)
  line L351 (78.0917, 45.6732) -> (78.092, 45.6732)
  line L352 (78.0917, 44.6481) -> (78.092, 44.6481)
  line L353 (78.092, 44.6481) -> (78.0917, 44.6481)
  circle A271 centre (78.0918, 42.6206) radius 1.0254
  arc A272 (78.0917, 43.1332) -> (78.0917, 42.1081) centre (78.0917, 42.6206) ccw
  arc A273 (78.092, 42.1081) -> (78.092, 43.1332) centre (78.092, 42.6206) ccw
  line L354 (78.0917, 43.1332) -> (78.092, 43.1332)
  line L355 (78.092, 43.1332) -> (78.0917, 43.1332)
  line L356 (78.092, 42.1081) -> (78.0917, 42.1081)
  line L357 (78.0917, 42.1081) -> (78.092, 42.1081)
  circle A274 centre (78.0918, 40.0806) radius 1.0254
  arc A275 (78.0917, 40.5932) -> (78.0917, 39.5681) centre (78.0917, 40.0806) ccw
  arc A276 (78.092, 39.5681) -> (78.092, 40.5932) centre (78.092, 40.0806) ccw
  line L358 (78.0917, 40.5932) -> (78.092, 40.5932)
  line L359 (78.092, 40.5932) -> (78.0917, 40.5932)
  line L360 (78.092, 39.5681) -> (78.0917, 39.5681)
  line L361 (78.0917, 39.5681) -> (78.092, 39.5681)
  circle A277 centre (78.0918, 37.5406) radius 1.0254
  arc A278 (78.0917, 38.0532) -> (78.0917, 37.0281) centre (78.0917, 37.5406) ccw
  arc A279 (78.092, 37.0281) -> (78.092, 38.0532) centre (78.092, 37.5406) ccw
  line L362 (78.092, 38.0532) -> (78.0917, 38.0532)
  line L363 (78.0917, 38.0532) -> (78.092, 38.0532)
  line L364 (78.0917, 37.0281) -> (78.092, 37.0281)
  line L365 (78.092, 37.0281) -> (78.0917, 37.0281)
  circle A280 centre (78.0847, 72.6655) radius 0.4732
  circle A281 centre (78.0847, 72.6655) radius 0.8383
  circle A282 centre (78.0847, 97.6657) radius 0.4732
  circle A283 centre (78.0847, 97.6657) radius 0.8383
  circle A284 centre (93.0849, 97.6657) radius 0.4732
  circle A285 centre (93.0849, 97.6657) radius 0.8383
  circle A286 centre (93.0849, 72.6655) radius 0.4732
  circle A287 centre (93.0849, 72.6655) radius 0.8383
  arc A288 (17.6311, 77.6725) -> (18.6645, 77.6725) centre (18.1478, 77.6725) ccw
  arc A289 (18.6645, 77.6728) -> (17.6311, 77.6728) centre (18.1478, 77.6728) ccw
  line L366 (17.6311, 77.6725) -> (17.6311, 77.6728)
  line L367 (17.6311, 77.6728) -> (17.6311, 77.6725)
  line L368 (18.6645, 77.6728) -> (18.6645, 77.6725)
  line L369 (18.6645, 77.6725) -> (18.6645, 77.6728)
  circle A290 centre (18.1478, 80.2126) radius 0.7794
  arc A291 (17.6311, 80.2125) -> (18.6645, 80.2125) centre (18.1478, 80.2125) ccw
  arc A292 (18.6645, 80.2128) -> (17.6311, 80.2128) centre (18.1478, 80.2128) ccw
  line L370 (17.6311, 80.2128) -> (17.6311, 80.2125)
  line L371 (17.6311, 80.2125) -> (17.6311, 80.2128)
  line L372 (18.6645, 80.2128) -> (18.6645, 80.2125)
  line L373 (18.6645, 80.2125) -> (18.6645, 80.2128)
  circle A293 centre (18.1478, 82.7526) radius 0.7794
  arc A294 (17.6311, 82.7525) -> (18.6645, 82.7525) centre (18.1478, 82.7525) ccw
  arc A295 (18.6645, 82.7528) -> (17.6311, 82.7528) centre (18.1478, 82.7528) ccw
  line L374 (17.6311, 82.7525) -> (17.6311, 82.7528)
  line L375 (17.6311, 82.7528) -> (17.6311, 82.7525)
  line L376 (18.6645, 82.7528) -> (18.6645, 82.7525)
  line L377 (18.6645, 82.7525) -> (18.6645, 82.7528)
  circle A296 centre (18.1478, 85.2926) radius 0.7794
  arc A297 (17.6311, 85.2925) -> (18.6645, 85.2925) centre (18.1478, 85.2925) ccw
  arc A298 (18.6645, 85.2928) -> (17.6311, 85.2928) centre (18.1478, 85.2928) ccw
  line L378 (17.6311, 85.2928) -> (17.6311, 85.2925)
  line L379 (17.6311, 85.2925) -> (17.6311, 85.2928)
  line L380 (18.6645, 85.2928) -> (18.6645, 85.2925)
  line L381 (18.6645, 85.2925) -> (18.6645, 85.2928)
  arc A299 (78.2443, 58.2395) -> (78.2443, 59.2598) centre (78.2443, 58.7496) ccw
  arc A300 (78.1933, 59.2598) -> (78.1933, 58.2395) centre (78.1933, 58.7496) ccw
  line L382 (78.1933, 58.2395) -> (78.2443, 58.2395)
  line L383 (78.2443, 58.2395) -> (78.1933, 58.2395)
  line L384 (78.2443, 59.2598) -> (78.1933, 59.2598)
  line L385 (78.1933, 59.2598) -> (78.2443, 59.2598)
  arc A301 (78.2443, 55.6995) -> (78.2443, 56.7198) centre (78.2443, 56.2096) ccw
  arc A302 (78.1933, 56.7198) -> (78.1933, 55.6995) centre (78.1933, 56.2096) ccw
  line L386 (78.2443, 55.6995) -> (78.1933, 55.6995)
  line L387 (78.1933, 55.6995) -> (78.2443, 55.6995)
  line L388 (78.2443, 56.7198) -> (78.1933, 56.7198)
  line L389 (78.1933, 56.7198) -> (78.2443, 56.7198)
  arc A303 (78.2443, 53.1595) -> (78.2443, 54.1798) centre (78.2443, 53.6696) ccw
  arc A304 (78.1933, 54.1798) -> (78.1933, 53.1595) centre (78.1933, 53.6696) ccw
  line L390 (78.1933, 53.1595) -> (78.2443, 53.1595)
  line L391 (78.2443, 53.1595) -> (78.1933, 53.1595)
  line L392 (78.1933, 54.1798) -> (78.2443, 54.1798)
  line L393 (78.2443, 54.1798) -> (78.1933, 54.1798)
  arc A305 (78.2443, 60.7795) -> (78.2443, 61.7998) centre (78.2443, 61.2896) ccw
  arc A306 (78.1933, 61.7998) -> (78.1933, 60.7795) centre (78.1933, 61.2896) ccw
  line L394 (78.1933, 60.7795) -> (78.2443, 60.7795)
  line L395 (78.2443, 60.7795) -> (78.1933, 60.7795)
  line L396 (78.2443, 61.7998) -> (78.1933, 61.7998)
  line L397 (78.1933, 61.7998) -> (78.2443, 61.7998)
  arc A307 (81.3711, 16.4798) -> (81.3711, 17.7515) centre (81.3711, 17.1156) ccw
  arc A308 (83.7026, 17.7515) -> (83.7026, 16.4798) centre (83.7026, 17.1156) ccw
  line L398 (83.7026, 16.4798) -> (81.3711, 16.4798)
  line L399 (81.3711, 16.4798) -> (83.7026, 16.4798)
  line L400 (83.7026, 17.7515) -> (81.3711, 17.7515)
  line L401 (81.3711, 17.7515) -> (83.7026, 17.7515)
  arc A309 (87.6727, 12.9877) -> (86.401, 12.9877) centre (87.0368, 12.9877) ccw
  arc A310 (86.401, 15.2435) -> (87.6727, 15.2435) centre (87.0368, 15.2435) ccw
  line L402 (86.401, 12.9877) -> (86.401, 15.2435)
  line L403 (86.401, 15.2435) -> (86.401, 12.9877)
  line L404 (87.6727, 12.9877) -> (87.6727, 15.2435)
  line L405 (87.6727, 15.2435) -> (87.6727, 12.9877)
  arc A311 (81.404, 9.8977) -> (81.404, 11.1336) centre (81.404, 10.5156) ccw
  arc A312 (83.6697, 11.1336) -> (83.6697, 9.8977) centre (83.6697, 10.5156) ccw
  line L406 (83.6697, 9.8977) -> (81.404, 9.8977)
  line L407 (81.404, 9.8977) -> (83.6697, 9.8977)
  line L408 (83.6697, 11.1336) -> (81.404, 11.1336)
  line L409 (81.404, 11.1336) -> (83.6697, 11.1336)
  circle A313 centre (83.9338, 61.6706) radius 0.4588
  circle A314 centre (83.9338, 59.1306) radius 0.4588
  circle A315 centre (83.9338, 59.1306) radius 0.8128
  circle A316 centre (83.9338, 56.5906) radius 0.4588
  circle A317 centre (83.9338, 56.5906) radius 0.8128
  circle A318 centre (83.9338, 54.0506) radius 0.4588
  circle A319 centre (83.9338, 54.0506) radius 0.8128
  circle A320 centre (46.4687, 53.4855) radius 0.35
  circle A321 centre (46.4688, 53.4857) radius 0.525
  circle A322 centre (46.4687, 54.7355) radius 0.35
  circle A323 centre (46.4688, 54.7357) radius 0.525
  circle A324 centre (46.4687, 55.9857) radius 0.35
  circle A325 centre (46.4688, 55.9858) radius 0.525
  circle A326 centre (46.4687, 57.2356) radius 0.35
  circle A327 centre (46.4688, 57.2358) radius 0.525
  circle A328 centre (46.4687, 58.4855) radius 0.35
  circle A329 centre (46.4688, 58.4857) radius 0.525
  circle A330 centre (46.4687, 59.7357) radius 0.35
  circle A331 centre (46.4688, 59.7359) radius 0.525
  circle A332 centre (46.4687, 60.9857) radius 0.35
  circle A333 centre (46.4688, 60.9858) radius 0.525
  circle A334 centre (46.4687, 62.2356) radius 0.35
  circle A335 centre (79.2348, 23.0626) radius 0.6
  circle A336 centre (79.2349, 25.6025) radius 0.6
  circle A337 centre (79.2348, 25.6026) radius 1
  circle A338 centre (79.2348, 28.1426) radius 0.6
  circle A339 centre (72.8849, 57.8696) radius 0.4572
  circle A340 centre (72.8848, 57.8695) radius 0.9525
  circle A341 centre (72.8849, 55.3296) radius 0.4572
  circle A342 centre (72.8848, 55.3295) radius 0.9525
  circle A343 centre (72.8849, 52.7896) radius 0.4572
  circle A344 centre (72.8848, 52.7895) radius 0.9525
  circle A345 centre (72.8849, 50.2496) radius 0.4572
  circle A346 centre (72.8848, 50.2495) radius 0.9525
  circle A347 centre (72.8849, 47.7096) radius 0.4572
  circle A348 centre (72.8848, 47.7095) radius 0.9525
  circle A349 centre (72.8849, 45.1696) radius 0.4572
  circle A350 centre (72.8848, 45.1695) radius 0.9525
  circle A351 centre (72.8849, 42.6296) radius 0.4572
  circle A352 centre (72.8848, 42.6295) radius 0.9525
  circle A353 centre (72.8849, 40.0896) radius 0.4572
  circle A354 centre (72.8848, 40.0895) radius 0.9525
  circle A355 centre (72.8849, 37.5496) radius 0.4572
  circle A356 centre (72.8848, 37.5495) radius 0.9525
  circle A357 centre (72.8849, 35.0096) radius 0.4572
  circle A358 centre (72.8848, 35.0095) radius 0.9525
  circle A359 centre (72.8849, 32.4696) radius 0.4572
  circle A360 centre (72.8848, 32.4695) radius 0.9525
  circle A361 centre (72.8849, 29.9296) radius 0.4572
  circle A362 centre (72.8848, 29.9295) radius 0.9525
  circle A363 centre (72.8849, 27.3896) radius 0.4572
  circle A364 centre (72.8848, 27.3895) radius 0.9525
  circle A365 centre (72.8849, 24.8496) radius 0.4572
  circle A366 centre (72.8848, 24.8495) radius 0.9525
  circle A367 centre (50.0249, 14.6896) radius 0.4572
  circle A368 centre (50.0248, 14.6895) radius 0.9525
  circle A369 centre (50.0249, 17.2296) radius 0.4572
  circle A370 centre (50.0248, 17.2295) radius 0.9525
  circle A371 centre (50.0249, 19.7696) radius 0.4572
  circle A372 centre (50.0248, 19.7695) radius 0.9525
  circle A373 centre (50.0249, 22.3096) radius 0.4572
  circle A374 centre (50.0248, 22.3095) radius 0.9525
  circle A375 centre (50.0249, 24.8496) radius 0.4572
  circle A376 centre (50.0248, 24.8495) radius 0.9525
  circle A377 centre (50.0249, 27.3896) radius 0.4572
  circle A378 centre (50.0248, 27.3895) radius 0.9525
  circle A379 centre (50.0249, 29.9296) radius 0.4572
  circle A380 centre (50.0248, 29.9295) radius 0.9525
  circle A381 centre (50.0249, 32.4696) radius 0.4572
  circle A382 centre (50.0248, 32.4695) radius 0.9525
  circle A383 centre (50.0249, 35.0096) radius 0.4572
  circle A384 centre (50.0248, 35.0095) radius 0.9525
  circle A385 centre (50.0249, 37.5496) radius 0.4572
  circle A386 centre (50.0248, 37.5495) radius 0.9525
  circle A387 centre (50.0249, 40.0896) radius 0.4572
  circle A388 centre (50.0248, 40.0895) radius 0.9525
  circle A389 centre (50.0249, 42.6296) radius 0.4572
  circle A390 centre (50.0248, 42.6295) radius 0.9525
  circle A391 centre (50.0249, 45.1696) radius 0.4572
  circle A392 centre (50.0248, 45.1695) radius 0.9525
  circle A393 centre (50.0249, 47.7096) radius 0.4572
  circle A394 centre (50.0248, 47.7095) radius 0.9525
  circle A395 centre (50.0249, 50.2496) radius 0.4572
  circle A396 centre (50.0248, 50.2495) radius 0.9525
  circle A397 centre (50.0249, 52.7896) radius 0.4572
  circle A398 centre (50.0248, 52.7895) radius 0.9525
  circle A399 centre (50.0249, 55.3296) radius 0.4572
  circle A400 centre (50.0248, 55.3295) radius 0.9525
  circle A401 centre (50.0249, 57.8696) radius 0.4572
  circle A402 centre (50.0248, 57.8695) radius 0.9525
  circle A403 centre (64.935, 66.4657) radius 0.4572
  circle A404 centre (64.9351, 66.4656) radius 0.762
  circle A405 centre (62.395, 66.4657) radius 0.4572
  circle A406 centre (62.3951, 66.4656) radius 0.762
  circle A407 centre (59.855, 66.4657) radius 0.4572
  circle A408 centre (59.8551, 66.4656) radius 0.762
  circle A409 centre (57.315, 66.4657) radius 0.4572
  circle A410 centre (57.3151, 66.4656) radius 0.762
  circle A411 centre (34.0228, 4.3936) radius 0.5
  circle A412 centre (34.0228, 4.3936) radius 1
  circle A413 centre (36.5628, 4.3936) radius 0.5
  circle A414 centre (36.5628, 4.3936) radius 1
  circle A415 centre (39.1028, 4.3936) radius 0.5
  circle A416 centre (39.1028, 4.3936) radius 1
  circle A417 centre (41.6428, 4.3936) radius 0.5
  circle A418 centre (41.6428, 4.3936) radius 1
  circle A419 centre (44.1828, 4.3936) radius 0.5
  circle A420 centre (44.1828, 4.3936) radius 1
  arc A421 (78.0917, 48.2005) -> (78.0917, 47.2007) centre (78.0917, 47.7006) ccw
  arc A422 (78.092, 47.2007) -> (78.092, 48.2005) centre (78.092, 47.7006) ccw
  line L410 (78.0917, 48.2005) -> (78.092, 48.2005)
  line L411 (78.092, 48.2005) -> (78.0917, 48.2005)
  line L412 (78.092, 47.2007) -> (78.0917, 47.2007)
  line L413 (78.0917, 47.2007) -> (78.092, 47.2007)
  circle A423 centre (78.0918, 45.1606) radius 1
  arc A424 (78.0917, 45.6605) -> (78.0917, 44.6607) centre (78.0917, 45.1606) ccw
  arc A425 (78.092, 44.6607) -> (78.092, 45.6605) centre (78.092, 45.1606) ccw
  line L414 (78.0917, 45.6605) -> (78.092, 45.6605)
  line L415 (78.092, 45.6605) -> (78.0917, 45.6605)
  line L416 (78.0917, 44.6607) -> (78.092, 44.6607)
  line L417 (78.092, 44.6607) -> (78.0917, 44.6607)
  circle A426 centre (78.0918, 42.6206) radius 1
  arc A427 (78.0917, 43.1205) -> (78.0917, 42.1207) centre (78.0917, 42.6206) ccw
  arc A428 (78.092, 42.1207) -> (78.092, 43.1205) centre (78.092, 42.6206) ccw
  line L418 (78.092, 43.1205) -> (78.0917, 43.1205)
  line L419 (78.0917, 43.1205) -> (78.092, 43.1205)
  line L420 (78.0917, 42.1207) -> (78.092, 42.1207)
  line L421 (78.092, 42.1207) -> (78.0917, 42.1207)
  circle A429 centre (78.0918, 40.0806) radius 1
  arc A430 (78.0917, 40.5805) -> (78.0917, 39.5807) centre (78.0917, 40.0806) ccw
  arc A431 (78.092, 39.5807) -> (78.092, 40.5805) centre (78.092, 40.0806) ccw
  line L422 (78.092, 40.5805) -> (78.0917, 40.5805)
  line L423 (78.0917, 40.5805) -> (78.092, 40.5805)
  line L424 (78.0917, 39.5807) -> (78.092, 39.5807)
  line L425 (78.092, 39.5807) -> (78.0917, 39.5807)
  circle A432 centre (78.0918, 37.5406) radius 1
  arc A433 (78.0917, 38.0405) -> (78.0917, 37.0407) centre (78.0917, 37.5406) ccw
  arc A434 (78.092, 37.0407) -> (78.092, 38.0405) centre (78.092, 37.5406) ccw
  line L426 (78.092, 38.0405) -> (78.0917, 38.0405)
  line L427 (78.0917, 38.0405) -> (78.092, 38.0405)
  line L428 (78.092, 37.0407) -> (78.0917, 37.0407)
  line L429 (78.0917, 37.0407) -> (78.092, 37.0407)
  circle A435 centre (78.0847, 72.6655) radius 0.4445
  circle A436 centre (78.0847, 72.6655) radius 0.7875
  circle A437 centre (78.0847, 97.6657) radius 0.4445
  circle A438 centre (78.0847, 97.6657) radius 0.7875
  circle A439 centre (93.0849, 97.6657) radius 0.4445
  circle A440 centre (93.0849, 97.6657) radius 0.7875
  circle A441 centre (93.0849, 72.6655) radius 0.4445
  circle A442 centre (93.0849, 72.6655) radius 0.7875
  arc A443 (17.648, 77.6725) -> (18.6477, 77.6725) centre (18.1478, 77.6725) ccw
  arc A444 (18.6477, 77.6727) -> (17.648, 77.6727) centre (18.1478, 77.6727) ccw
  line L430 (17.648, 77.6725) -> (17.648, 77.6727)
  line L431 (17.648, 77.6727) -> (17.648, 77.6725)
  line L432 (18.6477, 77.6725) -> (18.6477, 77.6727)
  line L433 (18.6477, 77.6727) -> (18.6477, 77.6725)
  circle A445 centre (18.1478, 80.2126) radius 0.754
  arc A446 (17.648, 80.2125) -> (18.6477, 80.2125) centre (18.1478, 80.2125) ccw
  arc A447 (18.6477, 80.2127) -> (17.648, 80.2127) centre (18.1478, 80.2127) ccw
  line L434 (17.648, 80.2127) -> (17.648, 80.2125)
  line L435 (17.648, 80.2125) -> (17.648, 80.2127)
  line L436 (18.6477, 80.2125) -> (18.6477, 80.2127)
  line L437 (18.6477, 80.2127) -> (18.6477, 80.2125)
  circle A448 centre (18.1478, 82.7526) radius 0.754
  arc A449 (17.648, 82.7525) -> (18.6477, 82.7525) centre (18.1478, 82.7525) ccw
  arc A450 (18.6477, 82.7527) -> (17.648, 82.7527) centre (18.1478, 82.7527) ccw
  line L438 (17.648, 82.7527) -> (17.648, 82.7525)
  line L439 (17.648, 82.7525) -> (17.648, 82.7527)